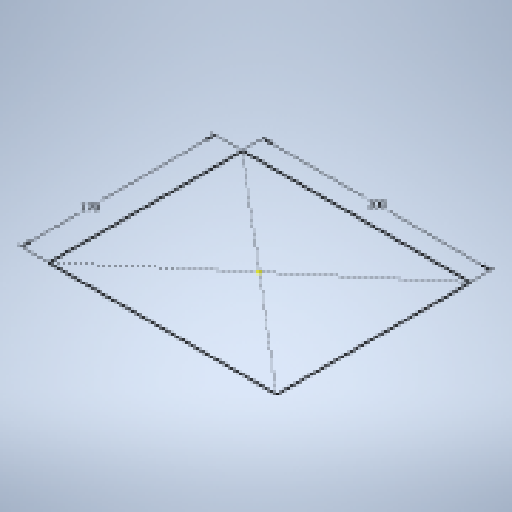
# Autodesk Inventor part: Base_Superior
Saved by Autodesk Inventor 2024 (Build 280153000, 153)
## iProperties
Created: 2025-05-14
Part Number: Base_Superior
Material: Genérico
Document SubType Name: Modeling
Designer: mario
Density: 1 g/cm^3
Appearance: Valor por defecto
Author: mario
Autodesk Inventor part; units mm, degrees
ref_plane "YZ Plane" through (0, 0, 0) normal (1, 0, 0) x (0, 1, 0)
ref_plane "XZ Plane" through (0, 0, 0) normal (0, 1, 0) x (-1, 0, 0)
ref_plane "XY Plane" through (0, 0, 0) normal (0, 0, 1) x (1, 0, 0)
sketch "Boceto1" plane through (0, 0, 0) normal (0, 1, 0) x (-1, 0, 0)
  line L0 (-100, 87.5) -> (100, 87.5)
  line L1 (100, 87.5) -> (100, -87.5)
  line L2 (100, -87.5) -> (-100, -87.5)
  line L3 (-100, -87.5) -> (-100, 87.5)
  line L4 (-100, 87.5) -> (100, -87.5) construction
  line L5 (100, 87.5) -> (-100, -87.5) construction
  point P0 (0, 0)
  dimension "d0" = 200
  dimension "d1" = 175
  constraints: 12 end point, 2 midpoint, 2 parallel, 1 horizontal, 1 perpendicular
  measures "d0" distance of L1.end L2.end
  measures "d1" distance of L0.end L1.end
extrude "Extrusión1" add sketch "Boceto1" along normal blind 3
fillet "Empalme1" radius 30 2 edges at (-100, 1.5, 87.5) (-100, 1.5, -87.5)
sketch "Boceto2" plane through (0, 3, 0) normal (0, 1, 0) x (1, 0, 0)
  line L0 (100, 87.5) -> (-70, 87.5) projected
  line L1 (-70, 87.5) -> (5, 87.5)
  line L2 (5, 87.5) -> (5, 68.5)
  line L3 (5, 68.5) -> (-70, 68.5)
  line L4 (-70, 68.5) -> (-70, 87.5)
  point P0 (0, 0)
  dimension "d5" = 75
  dimension "d6" = 19
  constraints: 8 end point, 2 parallel, 1 perpendicular, 1 point on line
  measures "d5" distance of L2.end L3.end
  measures "d6" distance of L1.end L2.end
extrude "Extrusión2" cut sketch "Boceto2" against normal blind 3
mirror "Simetría1" about plane through (0, 0, 0) normal (0, 0, 1) of "Extrusión2"
fillet "Empalme3" radius 5 8 edges at (-70, 1.5, -87.5) (-70, 1.5, -68.5) (5, 1.5, -87.5) (5, 1.5, -68.5) (5, 1.5, 87.5) (5, 1.5, 68.5) (-70, 1.5, 87.5) (-70, 1.5, 68.5)
sketch "Boceto3" plane through (0, 3, 0) normal (0, 1, 0) x (1, 0, 0)
  line L0 (-100, 57.5) -> (-100, -57.5) construction
  line L1 (-100, 0) -> (100, 0) construction
  line L2 (100, -87.5) -> (100, 87.5) construction
  point P0 (0, 0)
  point P1 (80, 15)
  point P2 (60, 15)
  point P3 (80, -15)
  point P4 (60, -15)
  dimension "d11" = 20
  dimension "d12" = 30
  dimension "d13" = 15
  dimension "d14" = 20
  constraints: 2 end point, 2 midpoint, 2 symmetric about line, 1 horizontal
  measures "d11" distance of point (60, 15) point (80, 15)
  measures "d12" distance of point (80, -15) point (80, 15)
  measures "d13" distance from line of L1 point (60, 15)
  measures "d14" distance from line of L2 point (80, 15)
hole "Agujero1" at (80, 3, -15) at (60, 3, -15) at (60, 3, 15) at (80, 3, 15) direction (0, -1, 0) diameter 2 end through all
sketch "Boceto5" plane through (0, 3, 0) normal (0, 1, 0) x (1, 0, 0)
  circle A0 centre (60, -15) radius 1 construction
  point P0 (0, 0)
  point P1 (70, 0)
  dimension "d22" = 15
  dimension "d23" = 10
  measures "d22" vertical distance of A0.centre point (70, 0)
  measures "d23" horizontal distance of A0.centre point (70, 0)
hole "Agujero2" at (70, 3, 0) direction (0, -1, 0) diameter 2.5 end through all
